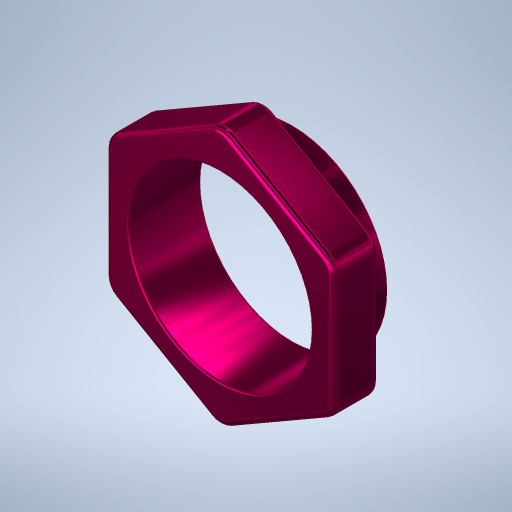
# Autodesk Inventor part: Shock Spring Adjustment Nut
Saved by Autodesk Inventor 2023.1 (Build 271208000, 208)
## iProperties
Created: 2019-11-29
Part Number: Shock Spring Adjustment Nut
Material: Generic
Document SubType Name: Modeling
Designer: Jopa
Density: 1 g/cm^3
Appearance: Anodized - Red
Author: Jopa
Autodesk Inventor part; units mm, degrees
ref_plane "YZ Plane" through (0, 0, 0) normal (1, 0, 0) x (0, 1, 0)
ref_plane "XZ Plane" through (0, 0, 0) normal (0, 1, 0) x (-1, 0, 0)
ref_plane "XY Plane" through (0, 0, 0) normal (0, 0, 1) x (1, 0, 0)
sketch "Sketch1" plane through (0, 0, 0) normal (0, 0, 1) x (1, 0, 0)
  circle A0 centre (0, 0) radius 6.6675
  dimension "d0" = 13.335
  constraints: 1 centre point, 1 coincident
  measures "d0" diameter of A0
extrude "Extrusion1" add sketch "Sketch1" along normal blind 1.905
sketch "Sketch2" plane through (0, 0, 1.905) normal (0, 0, 1) x (1, 0, 0)
  line L0 (-7.9375, 4.5827) -> (0, 9.1654)
  line L1 (0, 9.1654) -> (7.9375, 4.5827)
  line L2 (7.9375, 4.5827) -> (7.9375, -4.5827)
  line L3 (7.9375, -4.5827) -> (0, -9.1654)
  line L4 (0, -9.1654) -> (-7.9375, -4.5827)
  line L5 (-7.9375, -4.5827) -> (-7.9375, 4.5827)
  point P0 (0, 0)
  point P1 (0, 0)
  dimension "d3" = 15.875
  constraints: 12 end point, 1 coincident, 1 vertical, 13 other
  measures "d3" distance between parallel lines of L1 L4
extrude "Extrusion2" add sketch "Sketch2" along normal blind 3.175
sketch "Sketch3" plane through (0, 0, 0) normal (0, 0, -1) x (-1, 0, 0)
  circle A0 centre (0, 0) radius 6.35
  dimension "d6" = 12.7
  constraints: 1 centre point, 1 coincident
  measures "d6" diameter of A0
extrude "Extrusion3" cut sketch "Sketch3" against normal through all
fillet "Fillet1" radius 1.27 6 edges at (0, 9.1654, 3.4925) (7.9375, 4.5827, 3.4925) (7.9375, -4.5827, 3.4925) (0, -9.1654, 3.4925) (-7.9375, 4.5827, 3.4925) (-7.9375, -4.5827, 3.4925)
fillet "Fillet2" radius 0.381 24 edges at (7.7674, 4.4845, 1.905) (7.9375, 0, 1.905) (7.7674, -4.4845, 1.905) (3.9688, -6.8741, 1.905) (0, -8.969, 1.905) (-3.9687, -6.8741, 1.905) (-7.7674, -4.4845, 1.905) (-7.9375, 0, 1.905) (-7.7674, 4.4845, 1.905) (-3.9688, 6.8741, 1.905) (0, 8.969, 1.905) (3.9687, 6.8741, 1.905) (0, 8.969, 5.08) (-3.9688, 6.8741, 5.08) (-7.7674, 4.4845, 5.08) (-7.9375, 0, 5.08) (-7.7674, -4.4845, 5.08) (-3.9687, -6.8741, 5.08) (0, -8.969, 5.08) (3.9688, -6.8741, 5.08) (7.7674, -4.4845, 5.08) (7.9375, 0, 5.08) (7.7674, 4.4845, 5.08) (3.9687, 6.8741, 5.08)
fillet "Fillet3" radius 0.127 4 edges at (6.35, 0, 5.08) (-6.6675, 0, 1.905) (-6.6675, 0, 0) (6.35, 0, 0)
body "Solid1"
